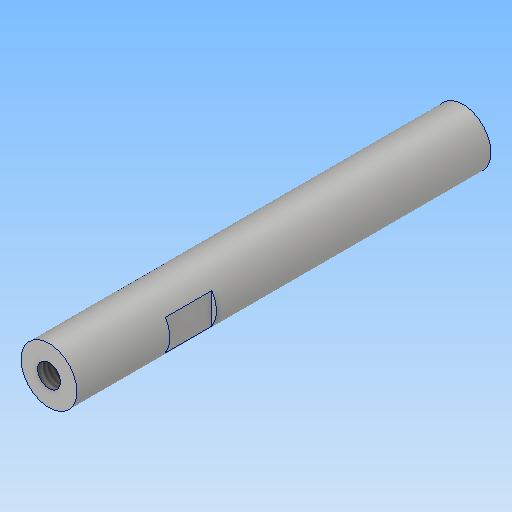
# Autodesk Inventor part: Pancake_Lever Weight
Saved by Autodesk Inventor 2018.1 (Build 221171000, 171)
## iProperties
Created: 2019-02-11
Part Number: Pancake_Lever Weight
Material: Aluminum 6061
Document SubType Name: Modeling
Designer: James
Density: 2.7 g/cm^3
Appearance: Aluminum - Flat
Mass: 3.13479 g
Surface Area: 10.3543 cm^2
Volume: 1.16103 cm^3
Author: James
Autodesk Inventor part; units mm, degrees
ref_plane "YZ Plane" through (0, 0, 0) normal (1, 0, 0) x (0, 1, 0)
ref_plane "XZ Plane" through (0, 0, 0) normal (0, 1, 0) x (-1, 0, 0)
ref_plane "XY Plane" through (0, 0, 0) normal (0, 0, 1) x (1, 0, 0)
sketch "Sketch1" plane through (0, 0, 0) normal (0, 0, 1) x (1, 0, 0)
  circle A0 centre (0, 0) radius 3
  dimension "d0" = 6
  constraints: 1 centre point, 1 coincident
  measures "d0" diameter of A0
extrude "Extrusion1" add sketch "Sketch1" along normal mid plane 44.5
sketch "Sketch2" plane through (0, 0, 22.25) normal (0, 0, 1) x (1, 0, 0)
  point P0 (0, 0)
  point P1 (0, 0)
  constraints: 1 coincident
hole "Hole1" at (0, 0, 22.25) direction (0, 0, -1) diameter 2.459 depth 8.8 tip angle 118 thread size "M3x0.5" class "6H" standard "ANSI Metric M Profile"
sketch "Sketch3" plane through (0, 0, 0) normal (0, 1, 0) x (-1, 0, 0)
  line L0 (3, 7.25) -> (2.5, 7.25)
  line L1 (2.5, 7.25) -> (2.5, 12.25)
  line L2 (2.5, 12.25) -> (3, 12.25)
  line L3 (3, 12.25) -> (3, 7.25)
  line L4 (-3, 12.25) -> (-2.5, 12.25)
  line L5 (-2.5, 12.25) -> (-2.5, 7.25)
  line L6 (-2.5, 7.25) -> (-3, 7.25)
  line L7 (-3, 7.25) -> (-3, 12.25)
  line L8 (-3, -22.25) -> (3, -22.25) projected
  line L9 (3, 22.25) -> (-3, 22.25) projected
  point P0 (0, 0)
  point P1 (-3, 23.75)
  dimension "d16" = 0.5
  dimension "d17" = 0.5
  dimension "d18" = 5
  dimension "d19" = 10
  constraints: 16 end point, 4 parallel, 2 horizontal, 2 horizontal alignment, 2 perpendicular, 2 vertical alignment, 1 point on line
  measures "d16" distance of L1.end L2.end
  measures "d17" distance of L4.start L4.end
  measures "d18" distance of L2.end L0.start
  measures "d19" distance between parallel lines of L9 L2
extrude "Extrusion2" cut sketch "Sketch3" along normal through all both and the other way through all
mirror "Mirror1" about plane through (0, 0, 0) normal (0, 0, 1) of "Hole1"
equation "\"d17\" = d16"
body "Solid1"
